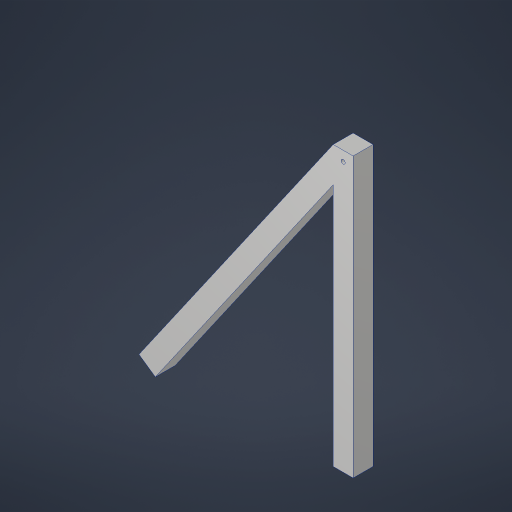
# Autodesk Inventor part: CL6-P1
Saved by Autodesk Inventor 2023.4 (Build 274418000, 418)
## iProperties
Created: 2025-03-16
Part Number: CL6-P1
Material: Aluminum 6061
Document SubType Name: Modeling
Designer: brand
Density: 2.7 g/cm^3
Appearance: Aluminum - Flat
Author: brand
Autodesk Inventor part; units mm, degrees
ref_plane "YZ Plane" through (0, 0, 0) normal (1, 0, 0) x (0, 1, 0)
ref_plane "XZ Plane" through (0, 0, 0) normal (0, 1, 0) x (-1, 0, 0)
ref_plane "XY Plane" through (0, 0, 0) normal (0, 0, 1) x (1, 0, 0)
sketch "Sketch1" plane through (0, 0, 0) normal (0, 0, 1) x (1, 0, 0)
  line L0 (0, 0) -> (-25.4, 0)
  line L1 (-25.4, 0) -> (-25.4, 355.6)
  line L2 (-25.4, 355.6) -> (0, 355.6)
  line L3 (0, 355.6) -> (0, 0)
  line L4 (-25.4, 355.6) -> (-273.05, 0)
  line L5 (-273.05, 0) -> (-252.2066, -14.5159)
  line L6 (-252.2066, -14.5159) -> (-4.5566, 341.0841)
  line L7 (-4.5566, 341.0841) -> (-25.4, 355.6)
  point P0 (-25.4, 311.1551)
  dimension "d0" = 25.4
  dimension "d1" = 355.6
  dimension "d2" = 25.4
  dimension "d3" = 273.05
  constraints: 16 end point, 4 parallel, 2 perpendicular, 1 horizontal, 1 horizontal alignment
  measures "d0" distance of L1.end L2.end
  measures "d1" distance of L0.end L1.end
  measures "d2" distance of L4.end L5.end
  measures "d3" distance of L0.start L4.end
extrude "Extrusion1" add sketch "Sketch1" against normal blind 25.4
sketch "Sketch2" plane through (0, 0, 0) normal (0, 0, 1) x (1, 0, 0)
  line L0 (0, 355.6) -> (0, 0) construction
  line L1 (0, 0) -> (-25.4, 0) construction
  line L2 (-25.4, 0) -> (-25.4, 311.1551) construction
  line L3 (-25.4, 311.1551) -> (-252.2066, -14.5159) construction
  line L4 (-252.2066, -14.5159) -> (-273.05, 0) construction
  line L5 (-273.05, 0) -> (-25.4, 355.6) construction
  line L6 (-25.4, 355.6) -> (0, 355.6) construction
  point P0 (-12.7, 342.9)
  dimension "d6" = 12.7
  dimension "d7" = 12.7
  measures "d6" distance from line of L6 point (-12.7, 342.9)
  measures "d7" distance from line of L0 point (-12.7, 342.9)
hole "Hole1" at (-12.7, 342.9, 0) direction (0, 0, -1) diameter 5.1054 end through all clearance for "Flat Head Machine Screw (82)" size "#10" standard "Ansi Unified Screw Threads"
equation "\"d2\" = d0"
equation "\"d7\" = d6"
body "Solid1"
